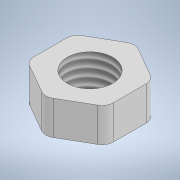
# Autodesk Inventor part: Moer
Saved by Autodesk Inventor 2022 (Build 260153000, 153)
## iProperties
Created: 2022-03-08
Part Number: Moer
Material: Generic
Document SubType Name: Modeling
Designer: 32497
Density: 1 g/cm^3
Appearance: Default
Author: 32497
Autodesk Inventor part; units mm, degrees
ref_plane "YZ Plane" through (0, 0, 0) normal (1, 0, 0) x (0, 1, 0)
ref_plane "XZ Plane" through (0, 0, 0) normal (0, 1, 0) x (-1, 0, 0)
ref_plane "XY Plane" through (0, 0, 0) normal (0, 0, 1) x (1, 0, 0)
sketch "Sketch1" plane through (0, 0, 0) normal (0, 1, 0) x (-1, 0, 0)
  circle A0 centre (0, 0) radius 2
  line L0 (3.5, -2.0207) -> (0, -4.0415)
  line L1 (0, -4.0415) -> (-3.5, -2.0207)
  line L2 (-3.5, -2.0207) -> (-3.5, 2.0207)
  line L3 (-3.5, 2.0207) -> (0, 4.0415)
  line L4 (0, 4.0415) -> (3.5, 2.0207)
  line L5 (3.5, 2.0207) -> (3.5, -2.0207)
  dimension "d0" = 4
  dimension "d1" = 3.5
  constraints: 12 end point, 2 coincident, 1 centre point, 13 other
  measures "d0" diameter of A0
  measures "d1" distance from line of point (0, 0) L5
extrude "Extrusion1" add sketch "Sketch1" along normal blind 3
thread "Thread1" size "M4x0.7" class "6H" standard "ANSI Metric M Profile" full length
fillet "Fillet1" radius 1 6 edges at (-3.5, 1.5, 2.0207) (0, 1.5, 4.0415) (3.5, 1.5, 2.0207) (3.5, 1.5, -2.0207) (0, 1.5, -4.0415) (-3.5, 1.5, -2.0207)
body "Solid1"
